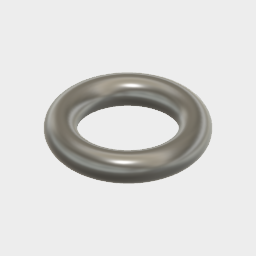
L10-PE-01 (Autodesk Fusion 360 design; units mm, degrees)
Autodesk Fusion 360 part; units mm, degrees
torus "TorusPrimitive1" add centre line diameter 100 section diameter 25 placed x (1, 0, 0) y (0, 0, -1) z (0, 1, 0) at (0, 0, 0)
